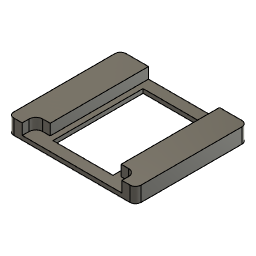
Display Spacer (Autodesk Fusion 360 design; units mm, degrees)
Autodesk Fusion 360 part; units mm, degrees
sketch "Sketch1" plane through (0, 0, 0) normal (0, 1, 0) x (1, 0, 0)
  line L0 (23.25, 20.5) -> (-23.25, 20.5)
  line L1 (-23.25, 20.5) -> (-23.25, -20.5)
  line L2 (-23.25, -20.5) -> (23.25, -20.5)
  line L3 (23.25, -20.5) -> (23.25, 20.5)
  line L4 (23.25, 20.5) -> (-23.25, -20.5) construction
  line L5 (-23.25, 20.5) -> (23.25, -20.5) construction
  dimension "d1" = 46.5
  dimension "d2" = 41
  constraint horizontal L0
  constraint perpendicular L0 L1
  constraint parallel L0 L2
  constraint parallel L1 L3
  constraint coincident L4 origin
  constraint coincident L5 origin
  measures "d1" distance of L1.end L2.end
  measures "d2" distance of L0.end L1.end
extrude "Extrude1" add sketch "Sketch1" along normal blind 5.5
sketch "Sketch2" plane through (0, 5.5, 0) normal (0, 1, 0) x (-1, 0, 0)
  line L0 (-23.25, 20.5) -> (-23.25, -20.5)
  line L1 (-23.25, -20.5) -> (23.25, -20.5)
  line L2 (23.25, -20.5) -> (23.25, 20.5)
  line L3 (23.25, 20.5) -> (-23.25, 20.5)
  line L4 (-13, -20.5) -> (13, -20.5)
  line L5 (13, -20.5) -> (13, 20.5)
  line L6 (13, 20.5) -> (-13, 20.5)
  line L7 (-13, 20.5) -> (-13, -20.5)
  line L8 (-13, -20.5) -> (13, 20.5) construction
  line L9 (13, -20.5) -> (-13, 20.5) construction
  line L10 (18.25, 20.5) -> (-18.25, 20.5)
  line L11 (-18.25, 20.5) -> (-18.25, 15.5)
  line L12 (-18.25, 15.5) -> (18.25, 15.5)
  line L13 (18.25, 15.5) -> (18.25, 20.5)
  dimension "d5" = 26
  dimension "d6" = 5
  dimension "d7" = 5
  dimension "d8" = 5
  constraint horizontal L4
  constraint perpendicular L4 L5
  constraint parallel L4 L6
  constraint parallel L5 L7
  constraint coincident L8 origin
  constraint coincident L9 origin
  constraint collinear L1 L4
  constraint horizontal L10
  constraint vertical L11
  constraint horizontal L12
  constraint vertical L13
  constraint coincident L3 L10.start
  measures "d5" distance of L5.end L6.end
  measures "d6" distance of L0 L11
  measures "d7" distance of L2 L13
  measures "d8" distance of L10 L12
extrude "Extrude2" cut sketch "Sketch2" against normal blind 4 contours L3 L7 L10 L11 L12 | L1 L4 L5 L7 L12 | L3 L5 L6 L7 L10 L12 | L3 L5 L10 L12 L13
fillet "Fillet1" radius 2.5 1 edges at (-18.25, 3.5, 15.5)
fillet "Fillet1" radius 2.5 1 edges at (18.25, 3.5, 15.5)
sketch "Sketch3" plane through (0, 1.5, 0) normal (0, 1, 0) x (-1, 0, 0)
  arc A0 (-18.25, 18) -> (-15.75, 15.5) centre (-15.75, 18) ccw
  line L0 (-15.75, 15.5) -> (-13, 15.5)
  line L1 (-13, 15.5) -> (-13, -20.5)
  line L2 (-13, -20.5) -> (13, -20.5)
  line L3 (13, -20.5) -> (13, 15.5)
  line L4 (13, 15.5) -> (15.75, 15.5)
  arc A1 (15.75, 15.5) -> (18.25, 18) centre (15.75, 18) ccw
  line L5 (18.25, 18) -> (18.25, 20.5)
  line L6 (18.25, 20.5) -> (-18.25, 20.5)
  line L7 (-18.25, 20.5) -> (-18.25, 18)
  line L8 (11, -16.5) -> (-11, -16.5)
  line L9 (-11, -16.5) -> (-11, 16.5)
  line L10 (-11, 16.5) -> (11, 16.5)
  line L11 (11, 16.5) -> (11, -16.5)
  dimension "d15" = 2
  dimension "d16" = 2
  dimension "d17" = 4
  dimension "d18" = 4
  constraint horizontal L8
  constraint vertical L9
  constraint horizontal L10
  constraint vertical L11
  measures "d15" distance of L3 L11
  measures "d16" distance of L1 L9
  measures "d17" distance of L2 L8
  measures "d18" distance of L6 L10
extrude "Extrude3" cut sketch "Sketch3" against normal blind 2 contours L8 L9 L10 L11
fillet "Fillet2" radius 2 tangency weight 1.28837 1 edges at (-23.25, 2.75, 20.5)
fillet "Fillet2" radius 2 1 edges at (23.25, 2.75, 20.5)
fillet "Fillet2" radius 2 1 edges at (23.25, 2.75, -20.5)
fillet "Fillet2" radius 2 1 edges at (-23.25, 2.75, -20.5)
